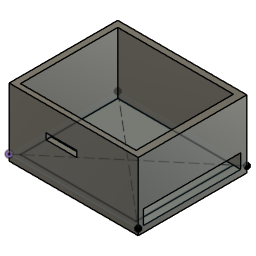
Box (Autodesk Fusion 360 design; units mm, degrees)
Autodesk Fusion 360 part; units mm, degrees
sketch "Dugnas" plane through (0, 0, 0) normal (0, 1, 0) x (1, 0, 0)
  line L0 (0, 0) -> (63, 0)
  line L1 (63, 0) -> (63, 53)
  line L2 (63, 53) -> (0, 53)
  line L3 (0, 53) -> (0, 0)
  dimension "d1" = 53
  dimension "d2" = 63
  constraint horizontal L0
  constraint vertical L1
  constraint horizontal L2
  constraint vertical L3
  constraint coincident L0.start L3.end
  measures "d1" distance of L0.start L2.end
  measures "d2" distance of L0.start L0.end
extrude "Extrude1" add sketch "Dugnas" along normal blind 3
sketch "Sienos" plane through (0, 3, 0) normal (0, 1, 0) x (-1, 0, 0)
  line L0 (0, -53) -> (0, 0)
  line L1 (0, 0) -> (-63, 0)
  line L2 (-63, 0) -> (-63, -53)
  line L3 (-63, -53) -> (0, -53)
  line L4 (0, 0) -> (-63, -53) construction
  line L5 (0, -53) -> (-63, 0) construction
  line L6 (-3, -2.5238) -> (-59.434, -2.5238)
  line L7 (-59.434, -2.5238) -> (-59.434, -50)
  line L8 (-59.434, -50) -> (-3, -50)
  line L9 (-3, -50) -> (-3, -2.5238)
  dimension "d5" = 3
  dimension "d6" = 3
  constraint coincident L0.end L1.start
  constraint coincident L2.end L3.start
  constraint coincident L0.start L3.end
  constraint coincident L1.end L2.start
  constraint horizontal L6
  constraint vertical L7
  constraint horizontal L8
  constraint vertical L9
  constraint coincident L4 L7.end
  constraint coincident L4 L6.start
  measures "d5" distance of L0 L9
  measures "d6" distance of L3 L8
extrude "Extrude4" add sketch "Sienos" along normal blind 30
sketch "USBC" plane through (59.434, 0, 0) normal (-1, 0, 0) x (0, 0, 1)
  line L0 (-50, 3) -> (-2.5238, 3)
  line L1 (-2.5238, 3) -> (-2.5238, 33)
  line L2 (-2.5238, 33) -> (-50, 33)
  line L3 (-50, 33) -> (-50, 3)
  line L4 (-50, 10) -> (0, 10)
  line L5 (-2.5238, 3) -> (-50, 3)
  dimension "d13" = 7
  constraint coincident L3 L4.start
  constraint perpendicular L1 L4
  measures "d13" distance of L4 L5
extrude "Extrude5" cut sketch "USBC" against normal blind 11 contours L0 L1 L3 L4 L5
sketch "LED" plane through (0, 0, -2.5238) normal (0, 0, -1) x (-1, 0, 0)
  line L0 (-63, 3) -> (-3, 3)
  line L1 (-3, 3) -> (-3, 33)
  line L2 (-3, 33) -> (-59.434, 33)
  line L3 (-59.434, 33) -> (-59.434, 10)
  line L4 (-59.434, 10) -> (-63, 10)
  line L5 (-63, 10) -> (-63, 3)
  line L6 (-18, 21) -> (-33, 21)
  line L7 (-33, 21) -> (-33, 18)
  line L8 (-33, 18) -> (-18, 18)
  line L9 (-18, 18) -> (-18, 21)
  line L10 (-3, 3) -> (-59.434, 3)
  point P0 (-63, 3)
  dimension "d16" = 15
  dimension "d17" = 3
  dimension "d18" = 30
  dimension "d19" = 15
  constraint horizontal L6
  constraint vertical L7
  constraint horizontal L8
  constraint vertical L9
  measures "d16" distance of L6.start L6.end
  measures "d17" distance of L6.end L7.end
  measures "d18" distance of L7 P0
  measures "d19" distance of L8 L10
extrude "Extrude6" cut sketch "LED" against normal blind 31 contours L6 L7 L8 L9
